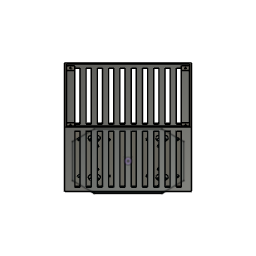
Quadrotor_controller_case v5 (Autodesk Fusion 360 design; units mm, degrees)
Autodesk Fusion 360 part; units mm, degrees
note: some values were not read from the file. Set by a fixed rule: the direction of a hole.
sketch "Sketch1" plane through (0, 0, 0) normal (0, 0, 1) x (1, 0, 0)
  line L0 (-15, -61.669) -> (15, -61.669)
  line L1 (15, -61.669) -> (61.669, -15)
  line L2 (61.669, -15) -> (61.669, 15)
  line L3 (61.669, 15) -> (15, 61.669)
  line L4 (15, 61.669) -> (-15, 61.669)
  line L5 (-15, 61.669) -> (-61.669, 15)
  line L6 (-61.669, 15) -> (-61.669, -15)
  line L7 (-61.669, -15) -> (-15, -61.669)
  dimension "d1" = 66
  dimension "d2" = 30
  dimension "d3" = 66
  dimension "d4" = 30
  dimension "d5" = 66
  dimension "d6" = 30
  dimension "d7" = 66
  dimension "d8" = 30
  dimension "d9" = 15
  dimension "d10" = 15
  dimension "d11" = 15
  dimension "d12" = 135
  constraint horizontal L0
  constraint perpendicular L0 L2
  constraint perpendicular L2 L4
  constraint perpendicular L4 L6
  measures "d1" distance of L0.start L6.end
  measures "d2" distance of L0.start L0.end
  measures "d3" distance of L0.end L1.end
  measures "d4" distance of L1.end L2.end
  measures "d5" distance of L2.end L3.end
  measures "d6" distance of L3.end L4.end
  measures "d7" distance of L4.end L5.end
  measures "d8" distance of L5.end L6.end
  measures "d9" horizontal distance of origin L3.end
  measures "d10" vertical distance of origin L2.end
  measures "d11" horizontal distance of origin L0.start
  measures "d12" angle of L3 L4
extrude "Extrude1" add sketch "Sketch1" along normal blind 2
sketch "Sketch4" plane through (0, 0, 2) normal (0, 0, 1) x (-1, 0, 0)
  line L0 (61.669, 15) -> (15, 61.669)
  line L1 (15, 61.669) -> (-15, 61.669)
  line L2 (-15, 61.669) -> (-61.669, 15)
  line L3 (-61.669, 15) -> (-61.669, -15)
  line L4 (-61.669, -15) -> (-15, -61.669)
  line L5 (-15, -61.669) -> (15, -61.669)
  line L6 (15, -61.669) -> (61.669, -15)
  line L7 (61.669, -15) -> (61.669, 15)
  line L8 (5.6306, 82.2108) -> (-82.0507, -5.4705)
  line L9 (-82.0507, -5.4705) -> (-5.4003, -82.1208)
  line L10 (-5.4003, -82.1208) -> (82.2809, 5.5604)
  line L11 (82.2809, 5.5604) -> (5.6306, 82.2108)
  line L12 (61.669, 15) -> (15, 61.669)
  dimension "d70" = 124
  dimension "d71" = 108.4
  dimension "d162" = 7.9
  constraint perpendicular L0 L8
  constraint perpendicular L8 L9
  constraint perpendicular L9 L10
  constraint perpendicular L8 L11
  measures "d70" distance of L8.start L8.end
  measures "d71" distance of L8.end L9.end
  measures "d162" distance of L11 L12
extrude "Extrude2" add sketch "Sketch4" along normal blind 2 contours L0 L1 L3 L4 L5 L6 L7 L8 L12 | L0 L1 L3 L4 L5 L6 L7 L8 L9 L10 L11 L12
sketch "Sketch6" plane through (0, 0, 4) normal (0, 0, 1) x (-1, 0, 0)
  line L0 (82.2809, 5.5604) -> (5.6306, 82.2108)
  line L1 (5.6306, 82.2108) -> (-82.0507, -5.4705)
  line L2 (-82.0507, -5.4705) -> (-5.4003, -82.1208)
  line L3 (-5.4003, -82.1208) -> (82.2809, 5.5604)
  line L4 (-82.0507, -5.4705) -> (-5.4003, -82.1208)
  line L5 (82.2809, 5.5604) -> (5.6306, 82.2108)
  line L6 (-79.2223, -5.4705) -> (-5.4003, -79.2924)
  line L7 (-5.4003, -79.2924) -> (79.4525, 5.5604)
  line L8 (79.4525, 5.5604) -> (5.6306, 79.3823)
  line L9 (5.6306, 79.3823) -> (-79.2223, -5.4705)
  dimension "d81" = 2
  dimension "d82" = 2
  dimension "d83" = 2
  dimension "d84" = 2
  constraint coincident L1.end L2.start
  constraint coincident L2.end L3.start
  constraint coincident L0.start L3.end
  constraint coincident L0.end L1.start
  constraint parallel L4 L6
  constraint perpendicular L6 L7
  constraint perpendicular L1 L8
  constraint perpendicular L6 L9
  measures "d81" distance of L4 L6
  measures "d82" distance of L3 L7
  measures "d83" distance of L5 L8
  measures "d84" distance of L1 L9
extrude "Extrude3" add sketch "Sketch6" along normal blind 75
sketch "Sketch7" plane through (38.2901, -38.2901, 0) normal (0.707107, -0.707107, 0) x (0.707107, 0.707107, 0)
  line L0 (-62.1132, 2) -> (-33.0628, 2)
  line L1 (61.8868, 2) -> (61.8868, 79)
  line L2 (61.8868, 79) -> (-62.1132, 79)
  line L3 (-62.1132, 79) -> (-62.1132, 2)
  line L4 (3, 7) -> (8, 7)
  line L5 (8, 7) -> (8, 74)
  line L6 (8, 74) -> (3, 74)
  line L7 (3, 74) -> (3, 7)
  line L8 (19, 7) -> (19, 74)
  line L9 (19, 74) -> (14, 74)
  line L10 (14, 74) -> (14, 7)
  line L11 (14, 7) -> (19, 7)
  line L12 (30, 7) -> (30, 74)
  line L13 (30, 74) -> (25, 74)
  line L14 (25, 74) -> (25, 7)
  line L15 (25, 7) -> (30, 7)
  line L16 (41, 7) -> (41, 74)
  line L17 (41, 74) -> (36, 74)
  line L18 (36, 74) -> (36, 7)
  line L19 (36, 7) -> (41, 7)
  line L20 (-3, 7) -> (-8, 7)
  line L21 (-8, 7) -> (-8, 74)
  line L22 (-8, 74) -> (-3, 74)
  line L23 (-3, 74) -> (-3, 7)
  line L24 (-19, 7) -> (-19, 74)
  line L25 (-14, 74) -> (-14, 7)
  line L26 (-14, 7) -> (-19, 7)
  line L27 (-19, 74) -> (-14, 74)
  line L28 (-30, 7) -> (-30, 74)
  line L29 (-25, 74) -> (-25, 7)
  line L30 (-25, 7) -> (-30, 7)
  line L31 (-30, 74) -> (-25, 74)
  line L32 (-41, 7) -> (-41, 74)
  line L33 (-36, 74) -> (-36, 7)
  line L34 (-36, 7) -> (-41, 7)
  line L35 (-41, 74) -> (-36, 74)
  line L36 (-52, 7) -> (-52, 74)
  line L37 (-47, 74) -> (-47, 7)
  line L38 (-47, 7) -> (-52, 7)
  line L39 (-52, 74) -> (-47, 74)
  line L40 (-33.0628, 2) -> (33.0628, 2)
  line L41 (33.0628, 2) -> (61.8868, 2)
  line L42 (52, 7) -> (52, 74)
  line L43 (52, 74) -> (47, 74)
  line L44 (47, 74) -> (47, 7)
  line L45 (47, 7) -> (52, 7)
  dimension "d89" = 44
  dimension "d90" = 0
  dimension "d93" = -44
  dimension "d94" = 0
  dimension "d177" = 5
  dimension "d178" = 3
  dimension "d179" = 3
  dimension "d180" = 5
  dimension "d181" = 5
  dimension "d182" = 5
  dimension "d183" = 5
  dimension "d184" = 5
  constraint horizontal L4
  constraint vertical L5
  constraint horizontal L6
  constraint vertical L7
  constraint horizontal L20
  constraint vertical L21
  constraint horizontal L22
  constraint vertical L23
  measures "d177" distance of L5.end L6.end
  measures "d178" horizontal distance of origin L4.start
  measures "d179" horizontal distance of origin L20.start
  measures "d180" distance of L21.end L22.end
  measures "d181" distance of L2 L36.end
  measures "d182" distance of L2 L42.end
  measures "d183" vertical distance of L0.end L33.end
  measures "d184" vertical distance of L1.start L42.start
extrude "Extrude4" cut sketch "Sketch7" against normal blind 150 contours L4 L5 L6 L7 | L8 L9 L10 L11 | L12 L13 L14 L15 | L16 L17 L18 L19 | L20 L21 L22 L23 | L24 L25 L26 L27 | L28 L29 L30 L31 | L32 L33 L34 L35 | L36 L37 L38 L39 | L42 L43 L44 L45
sketch "Sketch8" plane through (43.7606, 43.7606, 0) normal (0.707107, 0.707107, 0) x (-0.707107, 0.707107, 0)
  line L0 (-54.1504, 2) -> (54.2496, 2)
  line L1 (54.2496, 2) -> (54.2496, 79)
  line L2 (54.2496, 79) -> (-54.1504, 79)
  line L3 (-54.1504, 79) -> (-54.1504, 2)
  line L4 (3.5, 7) -> (9, 7)
  line L5 (9, 7) -> (9, 74)
  line L6 (9, 74) -> (3.5, 74)
  line L7 (3.5, 74) -> (3.5, 7)
  line L8 (20.6667, 7) -> (20.6667, 74)
  line L9 (20.6667, 74) -> (15.1667, 74)
  line L10 (15.1667, 74) -> (15.1667, 7)
  line L11 (15.1667, 7) -> (20.6667, 7)
  line L12 (32.3333, 7) -> (32.3333, 74)
  line L13 (32.3333, 74) -> (26.8333, 74)
  line L14 (26.8333, 74) -> (26.8333, 7)
  line L15 (26.8333, 7) -> (32.3333, 7)
  line L16 (44, 7) -> (44, 74)
  line L17 (44, 74) -> (38.5, 74)
  line L18 (38.5, 74) -> (38.5, 7)
  line L19 (38.5, 7) -> (44, 7)
  line L20 (-3.5, 7) -> (-9, 7)
  line L21 (-9, 7) -> (-9, 74)
  line L22 (-9, 74) -> (-3.5, 74)
  line L23 (-3.5, 74) -> (-3.5, 7)
  line L24 (-20.6667, 7) -> (-20.6667, 74)
  line L25 (-20.6667, 74) -> (-15.1667, 74)
  line L26 (-15.1667, 74) -> (-15.1667, 7)
  line L27 (-15.1667, 7) -> (-20.6667, 7)
  line L28 (-32.3333, 7) -> (-32.3333, 74)
  line L29 (-32.3333, 74) -> (-26.8333, 74)
  line L30 (-26.8333, 74) -> (-26.8333, 7)
  line L31 (-26.8333, 7) -> (-32.3333, 7)
  line L32 (-44, 7) -> (-44, 74)
  line L33 (-44, 74) -> (-38.5, 74)
  line L34 (-38.5, 74) -> (-38.5, 7)
  line L35 (-38.5, 7) -> (-44, 7)
  dimension "d99" = 35
  dimension "d100" = 0
  dimension "d103" = -35
  dimension "d104" = 0
  dimension "d185" = 5.5
  dimension "d186" = 5.5
  dimension "d187" = 5
  dimension "d188" = 5
  dimension "d189" = 5
  dimension "d190" = 5
  dimension "d191" = 3.5
  dimension "d192" = 3.5
  constraint horizontal L4
  constraint vertical L5
  constraint horizontal L6
  constraint vertical L7
  constraint horizontal L20
  constraint vertical L21
  constraint horizontal L22
  constraint vertical L23
  measures "d185" distance of L21.end L22.end
  measures "d186" distance of L5.end L6.end
  measures "d187" distance of L2 L32.end
  measures "d188" distance of L2 L16.end
  measures "d189" distance of L0 L32.start
  measures "d190" vertical distance of L0.end L16.start
  measures "d191" horizontal distance of origin L20.start
  measures "d192" horizontal distance of origin L4.start
extrude "Extrude5" cut sketch "Sketch8" against normal blind 150 contours L4 L5 L6 L7 | L8 L9 L10 L11 | L12 L13 L14 L15 | L16 L17 L18 L19 | L20 L21 L22 L23 | L24 L25 L26 L27 | L28 L29 L30 L31 | L32 L33 L34 L35
sketch "Sketch11" plane through (0, 0, 4) normal (0, 0, 1) x (-1, 0, 0)
  line L0 (-79.2223, -5.4705) -> (-5.4003, -79.2924)
  line L1 (-5.4003, -79.2924) -> (79.4525, 5.5604)
  line L2 (79.4525, 5.5604) -> (5.6306, 79.3823)
  line L3 (5.6306, 79.3823) -> (-79.2223, -5.4705)
  circle A0 centre (-8, 35.669) radius 1.5
  line L4 (15, 61.669) -> (-15, 61.669)
  circle A1 centre (8, 35.669) radius 1.5
  circle A2 centre (11.5, 55.669) radius 1.5
  circle A3 centre (-11.5, 55.669) radius 1.5
  point P0 (-35.669, -8)
  point P1 (-35.669, 8)
  point P2 (-55.669, 11.5)
  point P3 (-55.669, -11.5)
  point P4 (8, -35.669)
  point P5 (-8, -35.669)
  point P6 (-11.5, -55.669)
  point P7 (11.5, -55.669)
  point P8 (35.669, 8)
  point P9 (35.669, -8)
  point P10 (55.669, -11.5)
  point P11 (55.669, 11.5)
  dimension "d121" = 3
  dimension "d122" = 8
  dimension "d123" = 26
  dimension "d124" = 3
  dimension "d125" = 3
  dimension "d126" = 3
  dimension "d127" = 16
  dimension "d128" = 26
  dimension "d129" = 6
  dimension "d130" = 6
  dimension "d131" = 23
  dimension "d132" = 11.5
  dimension "d134" = 360
  measures "d121" diameter of A0
  measures "d122" horizontal distance of origin A0.centre
  measures "d123" distance of A0.centre L4
  measures "d124" diameter of A3
  measures "d125" diameter of A2
  measures "d126" diameter of A1
  measures "d127" horizontal distance of A0.centre A1.centre
  measures "d128" distance of L4 A1.centre
  measures "d129" distance of L4 A3.centre
  measures "d130" distance of L4 A2.centre
  measures "d131" distance of A2.centre A3.centre
  measures "d132" horizontal distance of origin A3.centre
hole "Hole12" at (11.5, -55.669, 4) at (-11.5, -55.669, 4) at (-8, -35.669, 4) at (8, -35.669, 4) at (-35.669, -8, 4) at (-55.669, -11.5, 4) at (-55.669, 11.5, 4) at (-35.669, 8, 4) at (-8, 35.669, 4) at (-11.5, 55.669, 4) at (11.5, 55.669, 4) at (8, 35.669, 4) at (55.669, 11.5, 4) at (35.669, 8, 4) at (35.669, -8, 4) at (55.669, -11.5, 4) direction (0, 0, -1) diameter 3 depth 15 tip angle 118 counterbore diameter 4.5 counterbore depth 2
sketch "Sketch12" plane through (0, 0, 0) normal (0, 0, 1) x (1, 0, 0)
  circle A0 centre (0, 31.669) radius 1.5
  circle A1 centre (-31.9699, 0) radius 1.5
  circle A2 centre (0, -31.669) radius 1.5
  circle A3 centre (31.9699, 0) radius 1.5
  line L0 (-15, -61.669) -> (15, -61.669)
  line L1 (15, 61.669) -> (-15, 61.669)
  dimension "d140" = 3
  dimension "d141" = 3
  dimension "d142" = 3
  dimension "d143" = 3
  dimension "d144" = 45
  dimension "d145" = 45
  dimension "d146" = 45
  dimension "d147" = 45
  dimension "d148" = 30
  dimension "d149" = 30
  measures "d140" diameter of A0
  measures "d141" diameter of A1
  measures "d142" diameter of A2
  measures "d143" diameter of A3
  measures "d144" distance of A0.centre A1.centre
  measures "d145" distance of A0.centre A3.centre
  measures "d146" distance of A2.centre A3.centre
  measures "d147" distance of A1.centre A2.centre
  measures "d148" distance of A2.centre L0
  measures "d149" distance of A0.centre L1
hole "Hole13" at (0, 31.669, 0) at (-31.9699, 0, 0) at (0, -31.669, 0) at (31.9699, 0, 0) direction (0, 0, 1) diameter 3 depth 15 tip angle 118 counterbore diameter 6 counterbore depth 2
sketch "Sketch13" plane through (0, 0, 4) normal (0, 0, 1) x (-1, 0, 0)
  circle A0 centre (0, 31.669) radius 1.5
  circle A1 centre (0, -31.669) radius 1.5
  circle A2 centre (31.9699, 0) radius 1.5
  circle A3 centre (-31.9699, 0) radius 1.5
  circle A4 centre (-35.669, 8) radius 2.25
  circle A5 centre (-55.669, -11.5) radius 2.25
  circle A6 centre (-11.5, -55.669) radius 2.25
  circle A7 centre (8, -35.669) radius 2.25
  circle A8 centre (55.669, -11.5) radius 2.25
  circle A9 centre (35.669, 8) radius 2.25
  circle A10 centre (8, 35.669) radius 2.25
  circle A11 centre (-11.5, 55.669) radius 2.25
  circle A12 centre (11.5, 55.669) radius 2.25
  circle A13 centre (-8, 35.669) radius 2.25
  circle A14 centre (55.669, 11.5) radius 2.25
  circle A15 centre (35.669, -8) radius 2.25
  circle A16 centre (11.5, -55.669) radius 2.25
  circle A17 centre (-8, -35.669) radius 2.25
  circle A18 centre (-35.669, -8) radius 2.25
  circle A19 centre (-55.669, 11.5) radius 2.25
  line L0 (-79.2223, -5.4705) -> (-5.4003, -79.2924)
  line L1 (-5.4003, -79.2924) -> (79.4525, 5.5604)
  line L2 (79.4525, 5.5604) -> (5.6306, 79.3823)
  line L3 (5.6306, 79.3823) -> (-79.2223, -5.4705)
  circle A20 centre (0.0237, -46.669) radius 6
  line L4 (-15, -61.669) -> (15, -61.669)
  circle A21 centre (46.669, 0.0237) radius 6
  circle A22 centre (-0.0237, 46.669) radius 6
  circle A23 centre (-46.669, -0.0237) radius 6
  dimension "d155" = 12
  dimension "d156" = 15
  dimension "d158" = 360
  measures "d155" diameter of A20
  measures "d156" distance of A20.centre L4
hole "Hole14" at (-0.0237, 46.669, 4) at (46.669, 0.0237, 4) at (0.0237, -46.669, 4) at (-46.669, -0.0237, 4) direction (0, 0, -1) diameter 12 depth 15 tip angle 118
sketch "Sketch14" plane through (0, 0, 4) normal (0, 0, 1) x (-1, 0, 0)
  circle A0 centre (-0.0237, 46.669) radius 6
  circle A1 centre (0.0237, -46.669) radius 6
  circle A2 centre (-46.669, -0.0237) radius 6
  circle A3 centre (46.669, 0.0237) radius 6
  circle A4 centre (0, 31.669) radius 1.5
  circle A5 centre (0, -31.669) radius 1.5
  circle A6 centre (31.9699, 0) radius 1.5
  circle A7 centre (-31.9699, 0) radius 1.5
  circle A8 centre (-35.669, 8) radius 2.25
  circle A9 centre (-55.669, -11.5) radius 2.25
  circle A10 centre (-11.5, -55.669) radius 2.25
  circle A11 centre (8, -35.669) radius 2.25
  circle A12 centre (55.669, -11.5) radius 2.25
  circle A13 centre (35.669, 8) radius 2.25
  circle A14 centre (8, 35.669) radius 2.25
  circle A15 centre (-11.5, 55.669) radius 2.25
  circle A16 centre (11.5, 55.669) radius 2.25
  circle A17 centre (-8, 35.669) radius 2.25
  circle A18 centre (55.669, 11.5) radius 2.25
  circle A19 centre (35.669, -8) radius 2.25
  circle A20 centre (11.5, -55.669) radius 2.25
  circle A21 centre (-8, -35.669) radius 2.25
  circle A22 centre (-35.669, -8) radius 2.25
  circle A23 centre (-55.669, 11.5) radius 2.25
  line L0 (-79.2223, -5.4705) -> (-5.4003, -79.2924)
  line L1 (-5.4003, -79.2924) -> (79.4525, 5.5604)
  line L2 (79.4525, 5.5604) -> (5.6306, 79.3823)
  line L3 (5.6306, 79.3823) -> (-79.2223, -5.4705)
  line L4 (79.4525, 5.5604) -> (73.7957, 11.2173)
  line L5 (73.7957, 11.2173) -> (68.1388, 5.5604)
  line L6 (68.1388, 5.5604) -> (73.7957, -0.0965)
  line L7 (79.4525, 5.5604) -> (73.7957, -0.0965)
  line L8 (-79.2223, -5.4705) -> (-73.5654, 0.1864)
  line L9 (-73.5654, 0.1864) -> (-67.9085, -5.4705)
  line L10 (-67.9085, -5.4705) -> (-73.5654, -11.1273)
  line L11 (-73.5654, -11.1273) -> (-79.2223, -5.4705)
  line L12 (5.6306, 79.3823) -> (11.2874, 73.7255)
  line L13 (11.2874, 73.7255) -> (5.6306, 68.0686)
  line L14 (5.6306, 68.0686) -> (-0.0263, 73.7255)
  line L15 (-0.0263, 73.7255) -> (5.6306, 79.3823)
  line L16 (-5.4003, -79.2924) -> (-11.0572, -73.6356)
  line L17 (-11.0572, -73.6356) -> (-5.4003, -67.9787)
  line L18 (-5.4003, -67.9787) -> (0.2565, -73.6356)
  line L19 (0.2565, -73.6356) -> (-5.4003, -79.2924)
  dimension "d163" = 8
  dimension "d164" = 8
  dimension "d167" = 8
  dimension "d168" = 8
  dimension "d171" = 8
  dimension "d172" = 8
  dimension "d173" = 8
  dimension "d174" = 8
  constraint coincident L1.end L2.start
  constraint coincident L2 L4.end
  constraint perpendicular L1 L4
  constraint perpendicular L4 L5
  constraint coincident L1 L6.end
  constraint perpendicular L1 L6
  constraint coincident L0.start L3.end
  constraint coincident L3 L8.end
  constraint perpendicular L0 L8
  constraint perpendicular L8 L9
  constraint coincident L0 L10.end
  constraint perpendicular L0 L10
  constraint coincident L2.end L3.start
  constraint coincident L2 L12.end
  constraint perpendicular L3 L12
  constraint perpendicular L12 L13
  constraint coincident L3 L14.end
  constraint perpendicular L3 L14
  constraint coincident L0.end L1.start
  constraint coincident L0 L16.end
  constraint perpendicular L16 L17
  constraint coincident L1 L18.end
  constraint perpendicular L1 L18
  constraint perpendicular L0 L19
  measures "d163" distance of L1.end L4.end
  measures "d164" distance of L6.end L1.end
  measures "d167" distance of L0.start L8.end
  measures "d168" distance of L10.end L0.start
  measures "d171" distance of L2.end L12.end
  measures "d172" distance of L2.end L14.end
  measures "d173" distance of L18.end L0.end
  measures "d174" distance of L0.end L16.end
extrude "Extrude6" add sketch "Sketch14" along normal blind 73 contours L0 L3 L8 L9 L10 L11 | L0 L1 L16 L17 L18 L19 | L2 L3 L12 L13 L14 L15 | L1 L2 L4 L5 L6 L7
sketch "Sketch16" plane through (0, 0, 77) normal (0, 0, 1) x (-1, 0, 0)
  line L0 (0.2565, -73.6356) -> (-5.4003, -67.9787)
  line L1 (-5.4003, -67.9787) -> (-11.0572, -73.6356)
  line L2 (-11.0572, -73.6356) -> (-5.4003, -79.2924)
  line L3 (-5.4003, -79.2924) -> (0.2565, -73.6356)
  circle A0 centre (-5.4003, -73.6356) radius 1
  circle A1 centre (73.7957, 5.5604) radius 1
  circle A2 centre (-73.5654, -5.4705) radius 1
  circle A3 centre (5.6306, 73.7255) radius 1
  line L4 (-5.4003, -79.2924) -> (-79.2223, -5.4705)
  line L5 (-79.2223, -5.4705) -> (5.6306, 79.3823)
  line L6 (5.6306, 79.3823) -> (79.4525, 5.5604)
  line L7 (79.4525, 5.5604) -> (-5.4003, -79.2924)
  dimension "d193" = 2
  dimension "d194" = 2
  dimension "d195" = 2
  dimension "d196" = 2
  dimension "d197" = 4
  dimension "d198" = 4
  dimension "d199" = 4
  dimension "d200" = 4
  dimension "d201" = 4
  dimension "d202" = 4
  dimension "d203" = 4
  dimension "d204" = 4
  measures "d193" diameter of A0
  measures "d194" diameter of A2
  measures "d195" diameter of A1
  measures "d196" diameter of A3
  measures "d197" distance of L1 A0.centre
  measures "d198" distance of L0 A0.centre
  measures "d199" distance of A2.centre L4
  measures "d200" distance of A2.centre L5
  measures "d201" distance of A3.centre L5
  measures "d202" distance of A3.centre L6
  measures "d203" distance of A1.centre L6
  measures "d204" distance of A1.centre L7
hole "Hole15" at (5.4003, 73.6356, 77) at (73.5654, 5.4705, 77) at (-5.6306, -73.7255, 77) at (-73.7957, -5.5604, 77) direction (0, 0, -1) diameter 2 depth 12 tip angle 118
sketch "Sketch17" plane through (-43.9207, -43.9207, 0) normal (-0.707107, -0.707107, 0) x (0.707107, -0.707107, 0)
  line L0 (-20.6667, 7) -> (-20.6667, 74)
  line L1 (-20.6667, 74) -> (-15.1667, 74)
  line L2 (-15.1667, 74) -> (-15.1667, 7)
  line L3 (-15.1667, 7) -> (-20.6667, 7)
  line L4 (26.8333, 74) -> (32.3333, 74)
  line L5 (32.3333, 74) -> (32.3333, 7)
  line L6 (32.3333, 7) -> (26.8333, 7)
  line L7 (26.8333, 7) -> (26.8333, 74)
  line L8 (15.1667, 74) -> (20.6667, 74)
  line L9 (20.6667, 74) -> (20.6667, 7)
  line L10 (20.6667, 7) -> (15.1667, 7)
  line L11 (15.1667, 7) -> (15.1667, 74)
  line L12 (-32.3333, 7) -> (-32.3333, 74)
  line L13 (-32.3333, 74) -> (-26.8333, 74)
  line L14 (-26.8333, 74) -> (-26.8333, 7)
  line L15 (-26.8333, 7) -> (-32.3333, 7)
  line L16 (-3.5, 7) -> (-9, 7)
  line L17 (-9, 7) -> (-9, 74)
  line L18 (-9, 74) -> (-3.5, 74)
  line L19 (-3.5, 74) -> (-3.5, 7)
  line L20 (38.5, 74) -> (44, 74)
  line L21 (44, 74) -> (44, 7)
  line L22 (44, 7) -> (38.5, 7)
  line L23 (38.5, 7) -> (38.5, 74)
  line L24 (9, 74) -> (9, 7)
  line L25 (9, 7) -> (3.5, 7)
  line L26 (3.5, 7) -> (3.5, 74)
  line L27 (3.5, 74) -> (9, 74)
  line L28 (-44, 7) -> (-44, 74)
  line L29 (-44, 74) -> (-38.5, 74)
  line L30 (-38.5, 74) -> (-38.5, 7)
  line L31 (-38.5, 7) -> (-44, 7)
  line L32 (-54.2496, 2) -> (54.1504, 2)
  line L33 (54.1504, 2) -> (54.1504, 79)
  line L34 (54.1504, 79) -> (-54.2496, 79)
  line L35 (-54.2496, 79) -> (-54.2496, 2)
  line L36 (-9, 7) -> (9, 7)
  line L37 (9, 7) -> (9, 30)
  line L38 (9, 30) -> (-9, 30)
  line L39 (-9, 30) -> (-9, 7)
  dimension "d208" = 23
  constraint horizontal L36
  constraint vertical L37
  constraint horizontal L38
  constraint vertical L39
  constraint coincident L24 L37.end
  constraint coincident L16.end L17.start
  measures "d208" distance of L16.end L38.end
extrude "Extrude7" add sketch "Sketch17" against normal blind 2 contours L16 L17 L19 L36 L38 L39 | L19 L26 L36 L38 | L24 L25 L26 L36 L37 L38
sketch "Sketch18" plane through (-43.9207, -43.9207, 0) normal (-0.707107, -0.707107, 0) x (0.707107, -0.707107, 0)
  line L0 (9, 30) -> (3.5, 30)
  line L1 (-6, 14) -> (9, 14)
  line L2 (9, 14) -> (9, 26)
  line L3 (9, 26) -> (-6, 26)
  line L4 (-6, 26) -> (-6, 14)
  line L5 (3.5, 30) -> (3.5, 74)
  line L6 (3.5, 74) -> (9, 74)
  line L7 (9, 74) -> (9, 30)
  line L8 (-3.5, 30) -> (-9, 30)
  line L9 (-9, 30) -> (-9, 74)
  line L10 (-9, 74) -> (-3.5, 74)
  line L11 (-3.5, 74) -> (-3.5, 30)
  line L12 (-20.6667, 7) -> (-20.6667, 74)
  line L13 (-20.6667, 74) -> (-15.1667, 74)
  line L14 (-15.1667, 74) -> (-15.1667, 7)
  line L15 (-15.1667, 7) -> (-20.6667, 7)
  line L16 (26.8333, 74) -> (32.3333, 74)
  line L17 (32.3333, 74) -> (32.3333, 7)
  line L18 (32.3333, 7) -> (26.8333, 7)
  line L19 (26.8333, 7) -> (26.8333, 74)
  line L20 (15.1667, 74) -> (20.6667, 74)
  line L21 (20.6667, 74) -> (20.6667, 7)
  line L22 (20.6667, 7) -> (15.1667, 7)
  line L23 (15.1667, 7) -> (15.1667, 74)
  line L24 (-32.3333, 7) -> (-32.3333, 74)
  line L25 (-32.3333, 74) -> (-26.8333, 74)
  line L26 (-26.8333, 74) -> (-26.8333, 7)
  line L27 (-26.8333, 7) -> (-32.3333, 7)
  line L28 (38.5, 74) -> (44, 74)
  line L29 (44, 74) -> (44, 7)
  line L30 (44, 7) -> (38.5, 7)
  line L31 (38.5, 7) -> (38.5, 74)
  line L32 (-44, 7) -> (-44, 74)
  line L33 (-44, 74) -> (-38.5, 74)
  line L34 (-38.5, 74) -> (-38.5, 7)
  line L35 (-38.5, 7) -> (-44, 7)
  line L36 (-54.2496, 2) -> (54.1504, 2)
  line L37 (54.1504, 2) -> (54.1504, 79)
  line L38 (54.1504, 79) -> (-54.2496, 79)
  line L39 (-54.2496, 79) -> (-54.2496, 2)
  dimension "d211" = 15
  dimension "d212" = 14
  dimension "d213" = 26
  dimension "d214" = 9
  constraint horizontal L1
  constraint vertical L2
  constraint horizontal L3
  constraint vertical L4
  measures "d211" distance of L1.start L1.end
  measures "d212" distance of origin L1
  measures "d213" distance of origin L3
  measures "d214" distance of origin L2
extrude "Extrude8" cut sketch "Sketch18" against normal blind 2 contours L1 L2 L3 L4
